Autodesk Fusion 360 part; units mm, degrees
(part 2 of 2)
sketch "Sketch25" plane through (0, 0, 0) normal (0, -1, 0) x (1, 0, 0)
  circle A0 centre (608.0806, 47.3768) radius 4
  circle A1 centre (290.245, 10.315) radius 1.632
  circle A2 centre (358.825, 49.685) radius 1.632
  circle A3 centre (290.245, 49.685) radius 1.632
  circle A4 centre (358.825, 10.315) radius 1.632
  line L0 (436.3768, 9) -> (436.3768, 7)
  line L1 (436.3768, 7) -> (431.3768, 7)
  line L2 (431.3768, 7) -> (431.3768, 9)
  line L3 (431.3768, 9) -> (436.3768, 9)
  line L4 (392.4, 53) -> (392.4, 51)
  line L5 (392.4, 51) -> (387.4, 51)
  line L6 (387.4, 51) -> (387.4, 53)
  line L7 (387.4, 53) -> (392.4, 53)
  line L8 (436.4, 53) -> (436.4, 51)
  line L9 (436.4, 51) -> (431.4, 51)
  line L10 (431.4, 51) -> (431.4, 53)
  line L11 (431.4, 53) -> (436.4, 53)
  line L12 (451.4, 22) -> (451.4, 17)
  line L13 (451.4, 17) -> (449.4, 17)
  line L14 (449.4, 17) -> (449.4, 22)
  line L15 (449.4, 22) -> (451.4, 22)
  line L16 (374.4, 22) -> (374.4, 17)
  line L17 (374.4, 17) -> (372.4, 17)
  line L18 (372.4, 17) -> (372.4, 22)
  line L19 (372.4, 22) -> (374.4, 22)
  line L20 (392.4, 7) -> (377.4, 7)
  line L21 (377.4, 7) -> (377.4, 47)
  arc A5 (378.4, 48) -> (377.4, 47) centre (378.4, 47) ccw
  line L22 (378.4, 48) -> (445.4, 48)
  arc A6 (446.4, 47) -> (445.4, 48) centre (445.4, 47) ccw
  line L23 (446.4, 47) -> (446.4, 13)
  arc A7 (445.4, 12) -> (446.4, 13) centre (445.4, 13) ccw
  line L24 (445.4, 12) -> (392.4, 12)
  line L25 (392.4, 12) -> (392.4, 7)
  line L26 (374.4, 43) -> (374.4, 38)
  line L27 (374.4, 38) -> (372.4, 38)
  line L28 (372.4, 38) -> (372.4, 43)
  line L29 (372.4, 43) -> (374.4, 43)
  line L30 (451.4, 43) -> (451.4, 38)
  line L31 (451.4, 38) -> (449.4, 38)
  line L32 (449.4, 38) -> (449.4, 43)
  line L33 (449.4, 43) -> (451.4, 43)
  line L34 (54.6452, 64.0786) -> (0.2658, 73.6672)
  arc A8 (0.2658, 73.6672) -> (15.4307, 51.4274) centre (30, 77.6521) ccw
  line L35 (15.4307, 51.4274) -> (47.2244, 33.7642)
  arc A9 (47.2244, 33.7642) -> (61.751, 29.989) centre (61.7937, 59.9889) ccw
  line L36 (61.751, 29.989) -> (121.5, 29.9038)
  arc A10 (121.5, 29.9038) -> (270.1218, 2.1743) centre (328.9822, 729.7974) ccw
  line L37 (270.1218, 2.1743) -> (297, 0)
  line L38 (297, 0) -> (481.4, 0)
  line L39 (481.4, 0) -> (481.4, 5)
  line L40 (481.4, 5) -> (486, 5)
  line L41 (486, 5) -> (486, 0)
  line L42 (486, 0) -> (638.7541, 27.9428)
  arc A11 (638.7541, 27.9428) -> (640.855, 36.8608) centre (637.8544, 32.8612) ccw
  line L43 (640.855, 36.8608) -> (618.013, 53.9974)
  arc A12 (618.013, 53.9974) -> (600.0096, 60) centre (600.0096, 30) ccw
  line L44 (600.0096, 60) -> (486, 60)
  line L45 (486, 60) -> (486, 55)
  line L46 (486, 55) -> (481.4, 55)
  line L47 (481.4, 55) -> (481.4, 60)
  line L48 (481.4, 60) -> (121.5429, 60)
  line L49 (121.5429, 60) -> (5.9649, 80.3795)
  arc A13 (5.9649, 80.3795) -> (0.931, 78.2208) centre (5.0967, 75.4555) ccw
  line L50 (0.931, 78.2208) -> (55.444, 68.6087)
  line L51 (55.444, 68.6087) -> (54.6452, 64.0786)
  line L52 (261, 60) -> (261, 2.9698)
  line L53 (270, 60) -> (274.6, 60)
  line L54 (274.6, 60) -> (274.6, 55)
  line L55 (274.6, 55) -> (270, 55)
  line L56 (270, 55) -> (270, 60)
  line L57 (247.4, 60) -> (252, 60)
  line L58 (252, 60) -> (252, 55)
  line L59 (252, 55) -> (247.4, 55)
  line L60 (247.4, 55) -> (247.4, 60)
  line L61 (224.8, 60) -> (229.4, 60)
  line L62 (229.4, 60) -> (229.4, 55)
  line L63 (229.4, 55) -> (224.8, 55)
  line L64 (224.8, 55) -> (224.8, 60)
  dimension "d204" = 225
  dimension "d205" = 5
  dimension "d206" = 4.6
  dimension "d207" = 9
  dimension "d208" = 9
  dimension "d209" = 18
  constraint coincident L48 L52.start
  constraint coincident A10 L52.end
  constraint perpendicular L48 L52
  constraint horizontal L53
  constraint vertical L54
  constraint horizontal L55
  constraint vertical L56
  constraint coincident L48 L53.start
  constraint horizontal L57
  constraint vertical L58
  constraint horizontal L59
  constraint vertical L60
  constraint coincident L48 L57.start
  constraint horizontal L61
  constraint vertical L62
  constraint horizontal L63
  constraint vertical L64
  constraint coincident L48 L61.start
  constraint equal L60 L62
  constraint equal L56 L60
  constraint equal L59 L63
  constraint equal L55 L59
  measures "d204" distance of L44.end L52.start
  measures "d205" distance of L61.start L63.end
  measures "d206" distance of L62.end L63.end
  measures "d207" distance of L52.start L53.start
  measures "d208" distance of L52.start L57.end
  measures "d209" distance of L57.start L61.end
extrude "Extrude14" cut sketch "Sketch25" against normal blind 10 contours L48 L61 L62 L63 L64 | L48 L57 L58 L59 L60 | L48 L53 L54 L55 L56
sketch "Sketch14" plane through (0, 0, 0) normal (0, -1, 0) x (1, 0, 0)
  circle A0 centre (608.0806, 47.3768) radius 4
  circle A1 centre (290.245, 10.315) radius 1.632
  circle A2 centre (358.825, 49.685) radius 1.632
  circle A3 centre (290.245, 49.685) radius 1.632
  circle A4 centre (358.825, 10.315) radius 1.632
  arc A5 (5.9649, 80.3795) -> (0.931, 78.2208) centre (5.0967, 75.4555) ccw
  arc A6 (0.2658, 73.6672) -> (15.4307, 51.4274) centre (30, 77.6521) ccw
  line L0 (15.4307, 51.4274) -> (47.2244, 33.7642)
  arc A7 (47.2244, 33.7642) -> (61.751, 29.989) centre (61.7937, 59.9889) ccw
  line L1 (61.751, 29.989) -> (121.5, 29.9038)
  arc A8 (121.5, 29.9038) -> (270.1218, 2.1743) centre (328.9822, 729.7974) ccw
  line L2 (270.1218, 2.1743) -> (297, 0)
  line L3 (297, 0) -> (481.4, 0)
  line L4 (481.4, 0) -> (481.4, 5)
  line L5 (481.4, 5) -> (486, 5)
  line L6 (486, 5) -> (486, 0)
  line L7 (486, 0) -> (638.7541, 27.9428)
  arc A9 (638.7541, 27.9428) -> (640.855, 36.8608) centre (637.8544, 32.8612) ccw
  line L8 (640.855, 36.8608) -> (618.013, 53.9974)
  arc A10 (618.013, 53.9974) -> (600.0096, 60) centre (600.0096, 30) ccw
  line L9 (600.0096, 60) -> (486, 60)
  line L10 (486, 60) -> (486, 55)
  line L11 (486, 55) -> (481.4, 55)
  line L12 (481.4, 55) -> (481.4, 60)
  line L13 (224.8, 60) -> (121.5429, 60)
  line L14 (121.5429, 60) -> (5.9649, 80.3795)
  line L15 (275.245, 44.697) -> (275.245, 13.8515)
  line L16 (146.3196, 50) -> (126.5286, 50)
  line L17 (126.5244, 47.0043) -> (126.5137, 39.5231)
  line L18 (145.6066, 31.7401) -> (196.4893, 23.3308)
  line L19 (121.5429, 60) -> (121.5, 29.9038)
  line L20 (275.245, 10.315) -> (290.245, 10.315)
  line L21 (77.8886, 34.966) -> (113.5071, 34.9152)
  line L22 (116.5114, 37.9109) -> (116.5245, 47.0988)
  line L23 (87.2027, 54.53) -> (28.389, 64.9004)
  line L24 (25.8981, 59.6835) -> (48.4796, 40.022)
  line L25 (54.2478, 30.9534) -> (54.2478, 71.8659)
  line L26 (15.4307, 51.4274) -> (15.4307, 78.7104)
  line L27 (496, 52) -> (496, 15.0573)
  line L28 (514.5755, 10.3102) -> (571.6338, 20.7477)
  line L29 (588.0806, 29.8203) -> (588.0806, 52)
  line L30 (588.0806, 55) -> (496, 55)
  line L31 (536.9832, 55) -> (499, 55)
  line L32 (544.4487, 55) -> (588.0806, 55)
  line L33 (290.245, 49.685) -> (345.825, 49.685)
  line L34 (358.825, 49.685) -> (358.825, 10.315)
  line L35 (358.825, 10.315) -> (303.245, 10.315)
  line L36 (290.245, 10.315) -> (290.245, 49.685)
  line L37 (315.5708, 49.4583) -> (348.825, 49.4583)
  line L38 (348.825, 46.685) -> (348.825, 17.6372)
  line L39 (334.6529, 10.0877) -> (300.245, 10.0877)
  line L40 (300.245, 13.315) -> (300.245, 43.0079)
  line L41 (130.7337, 36.7781) -> (147.5396, 44.2593)
  line L42 (144.7729, 37.3926) -> (163.7241, 46.7028)
  line L43 (166.5026, 46.6334) -> (198.4341, 28.9138)
  line L44 (179.9525, 44.4129) -> (215.683, 23.4364)
  line L45 (230.4442, 23.0758) -> (270.6997, 47.2684)
  line L46 (218.6893, 23.4182) -> (255.4279, 44.3948)
  line L47 (160.4357, 50) -> (170.4357, 50)
  line L48 (126.5071, 34.8967) -> (136.3733, 33.2661)
  line L49 (213.5872, 20.5051) -> (223.4534, 18.8745)
  line L50 (265.245, 50) -> (275.245, 50)
  line L51 (116.5071, 34.9109) -> (126.5071, 34.8967)
  line L52 (129.5244, 50) -> (160.4357, 50)
  line L53 (181.4714, 50) -> (253.9404, 50)
  line L54 (126.5071, 34.8967) -> (136.3733, 33.2661)
  line L55 (213.5872, 20.5051) -> (223.4534, 18.8745)
  line L56 (501.2833, 13.1114) -> (532.768, 50.0541)
  line L57 (511.7942, 15.2551) -> (541.0101, 48.0987)
  line L58 (554.2034, 49.6153) -> (583.2604, 27.4356)
  line L59 (545.1324, 48.4419) -> (572.9748, 26.0359)
  line L60 (496, 55) -> (530.4847, 55)
  line L61 (556.0237, 55) -> (585.0806, 55)
  line L62 (536.9832, 55) -> (547.1491, 55)
  line L63 (496, 6.9122) -> (506, 8.7415)
  line L64 (578.0806, 21.927) -> (588.0806, 23.7563)
  line L65 (112.7793, 50.009) -> (77.1477, 40.8719)
  line L66 (87.4269, 48.6696) -> (51.1948, 39.3785)
  line L67 (305.3143, 45.18) -> (336.7221, 15.2599)
  line L68 (313.5015, 44.2862) -> (343.7557, 15.465)
  arc A11 (28.389, 64.9004) -> (25.8981, 59.6835) centre (27.8681, 61.946) ccw
  arc A12 (48.4796, 40.022) -> (51.1948, 39.3785) centre (50.4496, 42.2845) ccw
  arc A13 (87.4269, 48.6696) -> (87.2027, 54.53) centre (86.6817, 51.5756) ccw
  arc A14 (77.1477, 40.8719) -> (77.8886, 34.966) centre (77.8929, 37.966) ccw
  arc A15 (116.5245, 47.0988) -> (112.7793, 50.009) centre (113.5245, 47.103) ccw
  arc A16 (113.5071, 34.9152) -> (116.5114, 37.9109) centre (113.5114, 37.9152) ccw
  arc A17 (129.5244, 50) -> (126.5244, 47.0043) centre (129.5244, 47) ccw
  arc A18 (126.5137, 39.5231) -> (130.7337, 36.7781) centre (129.5137, 39.5189) ccw
  arc A19 (147.5396, 44.2593) -> (146.3196, 50) centre (146.3196, 47) ccw
  arc A20 (166.5026, 46.6334) -> (163.7241, 46.7028) centre (165.047, 44.0102) ccw
  arc A21 (144.7729, 37.3926) -> (145.6066, 31.7401) centre (146.0957, 34.7) ccw
  arc A22 (196.4893, 23.3308) -> (198.4341, 28.9138) centre (196.9785, 26.2907) ccw
  arc A23 (181.4714, 50) -> (179.9525, 44.4129) centre (181.4714, 47) ccw
  arc A24 (215.683, 23.4364) -> (218.6893, 23.4182) centre (217.2018, 26.0235) ccw
  arc A25 (255.4279, 44.3948) -> (253.9404, 50) centre (253.9404, 47) ccw
  arc A26 (275.245, 44.697) -> (270.6997, 47.2684) centre (272.245, 44.697) ccw
  line L69 (231.5004, 17.5446) -> (271.7558, 10.8916)
  arc A27 (230.4442, 23.0758) -> (231.5004, 17.5446) centre (231.9895, 20.5045) ccw
  arc A28 (271.7558, 10.8916) -> (275.245, 13.8515) centre (272.245, 13.8515) ccw
  arc A29 (499, 55) -> (496, 52) centre (499, 52) ccw
  arc A30 (532.768, 50.0541) -> (530.4847, 55) centre (530.4847, 52) ccw
  arc A31 (496, 15.0573) -> (501.2833, 13.1114) centre (499, 15.0573) ccw
  arc A32 (545.1324, 48.4419) -> (541.0101, 48.0987) centre (543.2516, 46.1048) ccw
  arc A33 (511.7942, 15.2551) -> (514.5755, 10.3102) centre (514.0357, 13.2612) ccw
  arc A34 (556.0237, 55) -> (554.2034, 49.6153) centre (556.0237, 52) ccw
  arc A35 (588.0806, 52) -> (585.0806, 55) centre (585.0806, 52) ccw
  arc A36 (583.2604, 27.4356) -> (588.0806, 29.8203) centre (585.0806, 29.8203) ccw
  arc A37 (571.6338, 20.7477) -> (572.9748, 26.0359) centre (571.0939, 23.6987) ccw
  arc A38 (315.5708, 49.4583) -> (313.5015, 44.2862) centre (315.5708, 46.4583) ccw
  arc A39 (348.825, 46.685) -> (345.825, 49.685) centre (345.825, 46.685) ccw
  arc A40 (343.7557, 15.465) -> (348.825, 17.6372) centre (345.825, 17.6372) ccw
  arc A41 (334.6529, 10.0877) -> (336.7221, 15.2599) centre (334.6529, 13.0877) ccw
  arc A42 (300.245, 13.315) -> (303.245, 10.315) centre (303.245, 13.315) ccw
  arc A43 (305.3143, 45.18) -> (300.245, 43.0079) centre (303.245, 43.0079) ccw
  line L70 (436.3768, 9) -> (436.3768, 7)
  line L71 (436.3768, 7) -> (431.3768, 7)
  line L72 (431.3768, 7) -> (431.3768, 9)
  line L73 (431.3768, 9) -> (436.3768, 9)
  line L74 (392.4, 53) -> (392.4, 51)
  line L75 (392.4, 51) -> (387.4, 51)
  line L76 (387.4, 51) -> (387.4, 53)
  line L77 (387.4, 53) -> (392.4, 53)
  line L78 (436.4, 53) -> (436.4, 51)
  line L79 (436.4, 51) -> (431.4, 51)
  line L80 (431.4, 51) -> (431.4, 53)
  line L81 (431.4, 53) -> (436.4, 53)
  line L82 (451.4, 22) -> (451.4, 17)
  line L83 (451.4, 17) -> (449.4, 17)
  line L84 (449.4, 17) -> (449.4, 22)
  line L85 (449.4, 22) -> (451.4, 22)
  line L86 (374.4, 22) -> (374.4, 17)
  line L87 (374.4, 17) -> (372.4, 17)
  line L88 (372.4, 17) -> (372.4, 22)
  line L89 (372.4, 22) -> (374.4, 22)
  line L90 (392.4, 7) -> (377.4, 7)
  line L91 (377.4, 7) -> (377.4, 47)
  arc A44 (378.4, 48) -> (377.4, 47) centre (378.4, 47) ccw
  line L92 (378.4, 48) -> (445.4, 48)
  arc A45 (446.4, 47) -> (445.4, 48) centre (445.4, 47) ccw
  line L93 (446.4, 47) -> (446.4, 13)
  arc A46 (445.4, 12) -> (446.4, 13) centre (445.4, 13) ccw
  line L94 (445.4, 12) -> (392.4, 12)
  line L95 (392.4, 12) -> (392.4, 7)
  line L96 (374.4, 43) -> (374.4, 38)
  line L97 (374.4, 38) -> (372.4, 38)
  line L98 (372.4, 38) -> (372.4, 43)
  line L99 (372.4, 43) -> (374.4, 43)
  line L100 (451.4, 43) -> (451.4, 38)
  line L101 (451.4, 38) -> (449.4, 38)
  line L102 (449.4, 38) -> (449.4, 43)
  line L103 (449.4, 43) -> (451.4, 43)
  line L104 (54.6452, 64.0786) -> (0.2658, 73.6672)
  line L105 (0.931, 78.2208) -> (55.444, 68.6087)
  line L106 (55.444, 68.6087) -> (54.6452, 64.0786)
  line L107 (224.8, 55) -> (224.8, 60)
  line L108 (481.4, 60) -> (274.6, 60)
  line L109 (274.6, 60) -> (274.6, 55)
  line L110 (274.6, 55) -> (270, 55)
  line L111 (270, 55) -> (270, 60)
  line L112 (270, 60) -> (252, 60)
  line L113 (252, 60) -> (252, 55)
  line L114 (252, 55) -> (247.4, 55)
  line L115 (247.4, 55) -> (247.4, 60)
  line L116 (247.4, 60) -> (229.4, 60)
  line L117 (229.4, 60) -> (229.4, 55)
  line L118 (229.4, 55) -> (224.8, 55)
  dimension "d128" = 5
  dimension "d131" = 15
  dimension "d134" = 5
  dimension "d138" = 10
  dimension "d139" = 20
  dimension "d141" = 5
  dimension "d142" = 5
  dimension "d143" = 10
  dimension "d144" = 10
  dimension "d149" = 10
  dimension "d150" = 5
  dimension "d154" = 10
  dimension "d155" = 10
  dimension "d156" = 5
  dimension "d158" = 5
  dimension "d159" = 3
  dimension "d160" = 3
  dimension "d161" = 3
  dimension "d162" = 3
  dimension "d163" = 3
  dimension "d164" = 3
  dimension "d165" = 3
  dimension "d166" = 3
  dimension "d167" = 3
  dimension "d168" = 3
  dimension "d169" = 3
  dimension "d170" = 3
  dimension "d171" = 3
  dimension "d172" = 3
  dimension "d173" = 3
  dimension "d174" = 3
  dimension "d175" = 3
  dimension "d176" = 3
  dimension "d177" = 3
  dimension "d178" = 3
  dimension "d179" = 3
  dimension "d180" = 3
  dimension "d181" = 3
  dimension "d182" = 3
  dimension "d183" = 3
  dimension "d184" = 3
  dimension "d185" = 3
  dimension "d186" = 3
  dimension "d187" = 3
  dimension "d188" = 3
  dimension "d189" = 3
  dimension "d190" = 3
  dimension "d191" = 3
  constraint coincident L16 L47.start
  constraint coincident L13.end L14.start
  constraint coincident L1.end A8.start
  constraint parallel L17 L19
  constraint parallel L13 L16
  constraint coincident A1.centre L20.end
  constraint parallel L13 L20
  constraint parallel L19 L22
  constraint parallel L1 L21
  constraint midpoint A7 L25.start
  constraint coincident L14 L25.end
  constraint vertical L25
  constraint coincident A6.end L0.start
  constraint coincident L14 L26.end
  constraint vertical L26
  constraint parallel L12 L27
  constraint parallel L12 L29
  constraint perpendicular L27 L30
  constraint coincident L30 L31.start
  constraint perpendicular L29 L32
  constraint parallel L7 L28
  constraint horizontal L33
  constraint vertical L34
  constraint horizontal L35
  constraint vertical L36
  constraint coincident A4.centre L34.end
  constraint coincident A3.centre L33.start
  constraint horizontal L37
  constraint vertical L38
  constraint horizontal L39
  constraint vertical L40
  constraint coincident L18 L48.end
  constraint coincident L18 L49.start
  constraint coincident L18 L49.end
  constraint coincident L16 L50.start
  constraint horizontal L47
  constraint perpendicular L17 L51
  constraint perpendicular L15 L20
  constraint parallel L16 L53
  constraint equal L47 L50
  constraint equal L49 L50
  constraint parallel L48 L54
  constraint parallel L49 L55
  constraint equal L54 L55
  constraint coincident L28 L63.end
  constraint coincident L32 L62.end
  constraint coincident L28 L64.start
  constraint equal L62 L63
  constraint equal L63 L64
  constraint parallel L65 L66
  constraint parallel L67 L68
  constraint tangent L24 A11
  constraint tangent L23 A11
  constraint tangent L24 A12
  constraint tangent L66 A12
  constraint tangent L66 A13
  constraint tangent L23 A13
  constraint tangent L65 A14
  constraint tangent L21 A14
  constraint tangent L22 A15
  constraint tangent L65 A15
  constraint coincident L51.start L21
  constraint coincident L51.start L22
  constraint tangent L21 A16
  constraint tangent L22 A16
  constraint coincident L16.end L17
  constraint coincident L16.end L52
  constraint tangent L17 A17
  constraint tangent L52 A17
  constraint coincident L48.start L17
  constraint coincident L48.start L41
  constraint tangent L17 A18
  constraint tangent L41 A18
  constraint coincident L50.end L16
  constraint coincident L47.start L41
  constraint tangent L16 A19
  constraint tangent L41 A19
  constraint coincident L47.end L42
  constraint coincident L47.start L43
  constraint tangent L42 A20
  constraint tangent L43 A20
  constraint coincident L48.end L42
  constraint coincident L48.start L18
  constraint tangent L42 A21
  constraint tangent L18 A21
  constraint coincident L49.start L43
  constraint coincident L20.start L18
  constraint tangent L43 A22
  constraint tangent L18 A22
  constraint coincident L47.end L44
  constraint tangent L53 A23
  constraint tangent L44 A23
  constraint coincident L49.end L44
  constraint coincident L49.start L46
  constraint tangent L44 A24
  constraint tangent L46 A24
  constraint coincident L50.start L46
  constraint coincident L50.start L53
  constraint tangent L46 A25
  constraint tangent L53 A25
  constraint coincident L50.end L45
  constraint coincident L50.end L15
  constraint tangent L45 A26
  constraint tangent L15 A26
  constraint coincident L49.end L45
  constraint coincident L49.end L69
  constraint tangent L45 A27
  constraint tangent L69 A27
  constraint coincident L20.start L69
  constraint coincident L20.start L15
  constraint tangent L69 A28
  constraint tangent L15 A28
  constraint coincident L30.end L31
  constraint coincident L30.end L27
  constraint tangent L31 A29
  constraint tangent L27 A29
  constraint coincident L31.start L60
  constraint coincident L31.start L56
  constraint tangent L60 A30
  constraint tangent L56 A30
  constraint coincident L63.start L56
  constraint coincident L63.start L27
  constraint tangent L56 A31
  constraint tangent L27 A31
  constraint coincident L62.end L57
  constraint coincident L31.start L59
  constraint tangent L57 A32
  constraint tangent L59 A32
  constraint coincident L63.end L57
  constraint coincident L63.start L28
  constraint tangent L57 A33
  constraint tangent L28 A33
  constraint coincident L62.end L58
  constraint coincident L62.end L61
  constraint tangent L58 A34
  constraint tangent L61 A34
  constraint coincident L30.start L61
  constraint coincident L30.start L29
  constraint tangent L61 A35
  constraint tangent L29 A35
  constraint coincident L64.end L58
  constraint coincident L64.end L29
  constraint tangent L58 A36
  constraint tangent L29 A36
  constraint coincident L64.start L59
  constraint coincident L64.end L28
  constraint tangent L59 A37
  constraint tangent L28 A37
  constraint tangent L37 A38
  constraint tangent L68 A38
  constraint coincident A2.centre L33
  constraint coincident L37.end L38
  constraint tangent L33 A39
  constraint tangent L38 A39
  constraint tangent L68 A40
  constraint tangent L38 A40
  constraint tangent L67 A41
  constraint tangent L39 A41
  constraint coincident A1.centre L35
  constraint coincident L39.end L40
  constraint tangent L35 A42
  constraint tangent L40 A42
  constraint tangent L40 A43
  constraint tangent L67 A43
  measures "d128" distance of L17 L19
  measures "d131" distance of A3.centre L15
  measures "d134" distance of L19 L22
  measures "d138" distance of L10.end L27
  measures "d139" distance of A0.centre L29
  measures "d141" distance of L9 L30
  measures "d142" distance of L7 L28
  measures "d143" distance of L36 L40
  measures "d144" distance of L34 L38
  measures "d149" distance of L13 L16
  measures "d150" distance of L1.end L51
  measures "d154" distance of L48.start L48.end
  measures "d155" horizontal distance of L63.start L63.end
  measures "d156" distance of L65 L66
  measures "d158" distance of L67 L68
  measures "d159" radius of A11
  measures "d160" radius of A12
  measures "d161" radius of A13
  measures "d162" radius of A14
  measures "d163" radius of A15
  measures "d164" radius of A16
  measures "d165" radius of A17
  measures "d166" radius of A18
  measures "d167" radius of A19
  measures "d168" radius of A20
  measures "d169" radius of A21
  measures "d170" radius of A22
  measures "d171" radius of A23
  measures "d172" radius of A24
  measures "d173" radius of A25
  measures "d174" radius of A26
  measures "d175" radius of A27
  measures "d176" radius of A28
  measures "d177" radius of A29
  measures "d178" radius of A30
  measures "d179" radius of A31
  measures "d180" radius of A32
  measures "d181" radius of A33
  measures "d182" radius of A34
  measures "d183" radius of A35
  measures "d184" radius of A36
  measures "d185" radius of A37
  measures "d186" radius of A38
  measures "d187" radius of A39
  measures "d188" radius of A40
  measures "d189" radius of A41
  measures "d190" radius of A42
  measures "d191" radius of A43
extrude "Extrude11" cut sketch "Sketch14" against normal blind 20 contours L23 L24 L25 L66 A11 A12 | L23 L25 L66 A13 | L15 L45 A26 L69 A27 A28 | L16 L17 L41 L52 A17 A18 A19 | L18 L42 L43 A20 A21 A22 | L21 L22 L65 A14 A15 A16 | L27 L30 L31 L56 L60 A29 A30 A31 | L28 L57 L59 A32 A33 A37 | L29 L30 L32 L58 L61 A34 A35 A36 | L35 L40 L67 A41 A42 A43 | L37 L38 L68 A38 A39 A40 | L44 L46 L53 A23 A24 A25
ref_plane "WorkPlane1" through (121.5191, 2.25, 43.2708) normal (0.999999, 0, -0.001425) x (-0.001425, 0, -0.999999)
equation "d34 = ( 27 * 4.5 ) * 1 mm"
equation "d37 = ( 27 * 11 ) * 1 mm"
equation "d38 = ( 27 * 18 ) * 1 mm"

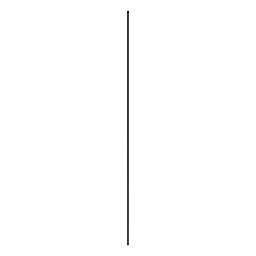
design "small spar short"
Autodesk Fusion 360 part; units mm, degrees
sketch "Sketch1" plane through (0, 0, 0) normal (0, 0, 1) x (1, 0, 0)
  circle A0 centre (0, 0) radius 1
  dimension "d1" = 2
  constraint coincident A0.centre origin
  measures "d1" diameter of A0
extrude "Extrude1" add sketch "Sketch1" along normal blind 322

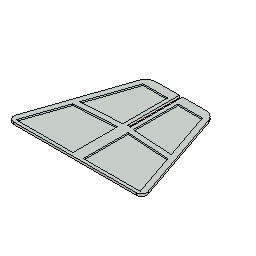
design "Tail Wing"
Autodesk Fusion 360 part; units mm, degrees
sketch "Sketch1" plane through (0, 0, 0) normal (0, 0, 1) x (1, 0, 0)
  line L0 (0, 0) -> (120, 0)
  line L1 (120, 0) -> (120, 120)
  line L2 (120, 120) -> (0, 120)
  line L3 (0, 120) -> (0, 0)
  dimension "d1" = 120
  constraint horizontal L0
  constraint vertical L1
  constraint horizontal L2
  constraint vertical L3
  constraint coincident L0.start L3.end
  constraint equal L0 L3
  measures "d1" distance of L1 L3
sketch "Sketch2" plane through (0, 0, 0) normal (0, 0, 1) x (1, 0, 0)
  line L0 (120.1825, 14.3012) -> (85.1178, 116.8012)
  line L1 (85.1178, 116.8012) -> (58.9029, 116.8012)
  line L2 (58.9029, 116.8012) -> (58.9029, 14.3012)
  line L3 (58.9029, 14.3012) -> (120.1825, 14.3012)
  line L4 (58.9029, 108.8012) -> (82.5701, 108.8012)
  line L5 (82.5701, 108.8012) -> (113.8718, 17.3012)
  line L6 (113.8718, 17.3012) -> (58.9029, 17.3012)
  line L7 (98.2209, 63.0512) -> (58.9029, 65.5512)
  line L8 (99.9346, 58.042) -> (58.9029, 60.6509)
  line L9 (58.9029, 116.8012) -> (48.9029, 116.8012)
  line L10 (48.9029, 116.8012) -> (48.9029, 14.3012)
  line L11 (48.9029, 14.3012) -> (58.9029, 14.3012)
  line L12 (58.9029, 14.3012) -> (58.9029, 116.8012)
  line L13 (53.9029, 116.8012) -> (53.9029, 14.3012)
  line L14 (48.9029, 108.8012) -> (25.2358, 108.8012)
  line L15 (22.6881, 116.8012) -> (48.9029, 116.8012)
  line L16 (-12.3766, 14.3012) -> (22.6881, 116.8012)
  line L17 (25.2358, 108.8012) -> (-6.0659, 17.3012)
  line L18 (9.585, 63.0512) -> (48.9029, 65.5512)
  line L19 (7.8713, 58.042) -> (48.9029, 60.6509)
  line L20 (-6.0659, 17.3012) -> (48.9029, 17.3012)
  line L21 (48.9029, 14.3012) -> (-12.3766, 14.3012)
  line L22 (48.9029, 14.3012) -> (48.9029, 116.8012)
  line L23 (58.9029, 14.3012) -> (48.9029, 14.3012)
  line L24 (48.9029, 116.8012) -> (58.9029, 116.8012)
  line L25 (48.9029, 17.3012) -> (48.9029, 14.3012)
  point P0 (120.1825, 14.3012)
  point P1 (53.9029, 14.3012)
  dimension "d2" = 3
  dimension "d3" = 5
  dimension "d4" = 8
  dimension "d5" = 10
  dimension "d18" = 102.5
  constraint coincident P0 L0.start
  constraint horizontal L1
  constraint perpendicular L1 L2
  constraint perpendicular L2 L3
  constraint coincident L2 L4.start
  constraint perpendicular L2 L4
  constraint parallel L0 L5
  constraint coincident L2 L6.end
  constraint perpendicular L2 L6
  constraint midpoint L5 L7.start
  constraint midpoint L2 L7.end
  constraint coincident L5 L8.start
  constraint coincident L2 L8.end
  constraint parallel L7 L8
  constraint horizontal L9
  constraint vertical L10
  constraint horizontal L11
  constraint vertical L12
  constraint midpoint L9 L13.start
  constraint midpoint L11 P1
  constraint symmetric P0 L13 L16.start
  constraint symmetric L0.end L13 L15.start
  constraint symmetric L1.end L13 L9.end
  constraint symmetric L2.end L13 L10.end
  constraint symmetric L4.start L13 L14.start
  constraint symmetric L4.end L13 L14.end
  constraint symmetric L5.end L13 L17.end
  constraint symmetric L6.end L13 L20.end
  constraint symmetric L7.start L13 L18.start
  constraint symmetric L7.end L13 L18.end
  constraint symmetric L8.start L13 L19.start
  constraint symmetric L8.end L13 L19.end
  constraint symmetric L9.end L13 L1.end
  constraint symmetric L10.end L13 L2.end
  constraint symmetric P1 L13 L13.end
  constraint coincident L10.end L11.start
  measures "d2" distance of L3 L6
  measures "d3" distance of L0 L5
  measures "d4" distance of L1 L4
  measures "d5" distance of L10 L12
  measures "d18" distance of L15 L21
extrude "Extrude1" add sketch "Sketch2" along normal blind 3.175 contours L0 L1 L2 L3 L4 L5 L6 L12 | L2 L9 L11 L12 L13 L23 L24 | L9 L10 L11 L13 L22 L23 L24 L25 | L2 L5 L7 L8 L12 | L10 L14 L15 L16 L17 L20 L21 L22 L25 | L10 L17 L18 L19 L22
extrude "Extrude2" add sketch "Sketch2" along normal blind 1 contours L2 L5 L6 L8 L12 | L2 L4 L5 L7 L12 | L10 L17 L19 L20 L22 | L10 L14 L17 L18 L22
fillet "Fillet1" radius 10 1 edges at (85.1178, 116.8012, 1.5875)
fillet "Fillet2" radius 10 1 edges at (22.6881, 116.8012, 1.5875)
fillet "Fillet3" radius 5 1 edges at (120.1825, 14.3012, 1.5875)
fillet "Fillet5" radius 5 1 edges at (-12.3766, 14.3012, 1.5875)
scale "Scale1" factors (1.5, 1.5, 1) about (48.9029, 65.5512, 1) bodies 1
sketch "Sketch5" plane through (0, 0, 3.175) normal (0, 0, 1) x (-1, 0, 0)
  arc A0 (39.6202, 1.3962) -> (32.524, 11.3238) centre (32.524, 3.8238) ccw
  line L0 (32.524, 11.3238) -> (-145.3299, 11.3238)
  arc A1 (-145.3299, 11.3238) -> (-152.4261, 1.3962) centre (-145.3299, 3.8238) ccw
  line L1 (-152.4261, 1.3962) -> (-106.6957, -132.2814)
  arc A2 (-106.6957, -132.2814) -> (-92.5032, -142.4262) centre (-92.5032, -127.4262) ccw
  line L2 (-92.5032, -142.4262) -> (-20.3027, -142.4262)
  arc A3 (-20.3027, -142.4262) -> (-6.1102, -132.2814) centre (-20.3027, -127.4262) ccw
  line L3 (-6.1102, -132.2814) -> (39.6202, 1.3962)
  line L4 (-99.4036, -130.4262) -> (-122.8799, -61.8012)
  line L5 (-122.8799, -61.8012) -> (-63.9029, -65.5512)
  line L6 (-63.9029, -65.5512) -> (-63.9029, -130.4262)
  line L7 (-63.9029, -130.4262) -> (-99.4036, -130.4262)
  line L8 (33.5503, 6.8238) -> (12.6445, -54.2873)
  line L9 (12.6445, -54.2873) -> (-48.9029, -58.2008)
  line L10 (-48.9029, -58.2008) -> (-48.9029, 6.8238)
  line L11 (-48.9029, 6.8238) -> (33.5503, 6.8238)
  line L12 (-63.9029, -58.2008) -> (-125.4504, -54.2873)
  line L13 (-125.4504, -54.2873) -> (-146.3562, 6.8238)
  line L14 (-146.3562, 6.8238) -> (-63.9029, 6.8238)
  line L15 (-63.9029, 6.8238) -> (-63.9029, -58.2008)
  line L16 (-48.9029, -65.5512) -> (10.074, -61.8012)
  line L17 (10.074, -61.8012) -> (-13.4023, -130.4262)
  line L18 (-13.4023, -130.4262) -> (-48.9029, -130.4262)
  line L19 (-48.9029, -130.4262) -> (-48.9029, -65.5512)
  line L20 (-54.1029, -142.4262) -> (-58.7029, -142.4262)
  line L21 (-58.7029, -142.4262) -> (-58.7029, -67.4262)
  line L22 (-58.7029, -67.4262) -> (-54.1029, -67.4262)
  line L23 (-54.1029, -67.4262) -> (-54.1029, -142.4262)
  line L24 (-54.1029, -132.8434) -> (-48.9029, -132.8434)
  line L25 (-58.7029, -133.3407) -> (-63.9029, -133.3407)
  dimension "d28" = 4.6
  dimension "d29" = 75
  constraint horizontal L20
  constraint vertical L21
  constraint horizontal L22
  constraint vertical L23
  constraint coincident L2 L20.start
  constraint coincident L23 L24.start
  constraint coincident L19 L24.end
  constraint perpendicular L19 L24
  constraint coincident L21 L25.start
  constraint coincident L6 L25.end
  constraint perpendicular L6 L25
  constraint equal L24 L25
  measures "d28" distance of L21 L23
  measures "d29" distance of L20.start L22.end
extrude "Extrude4" cut sketch "Sketch5" against normal blind 10 contours L2 L20 L21 L22 L23
sketch "Sketch7" plane through (0, 0, 3.175) normal (0, 0, 1) x (-1, 0, 0)
  line L0 (-54.1029, -67.4262) -> (-54.1029, -142.4262)
  line L1 (-54.1029, -142.4262) -> (-20.3027, -142.4262)
  arc A0 (-20.3027, -142.4262) -> (-6.1102, -132.2814) centre (-20.3027, -127.4262) ccw
  line L2 (-6.1102, -132.2814) -> (39.6202, 1.3962)
  arc A1 (39.6202, 1.3962) -> (32.524, 11.3238) centre (32.524, 3.8238) ccw
  line L3 (32.524, 11.3238) -> (-145.3299, 11.3238)
  arc A2 (-145.3299, 11.3238) -> (-152.4261, 1.3962) centre (-145.3299, 3.8238) ccw
  line L4 (-152.4261, 1.3962) -> (-106.6957, -132.2814)
  arc A3 (-106.6957, -132.2814) -> (-92.5032, -142.4262) centre (-92.5032, -127.4262) ccw
  line L5 (-92.5032, -142.4262) -> (-58.7029, -142.4262)
  line L6 (-58.7029, -142.4262) -> (-58.7029, -67.4262)
  line L7 (-58.7029, -67.4262) -> (-54.1029, -67.4262)
  line L8 (-99.4036, -130.4262) -> (-122.8799, -61.8012)
  line L9 (-122.8799, -61.8012) -> (-63.9029, -65.5512)
  line L10 (-63.9029, -65.5512) -> (-63.9029, -130.4262)
  line L11 (-63.9029, -130.4262) -> (-99.4036, -130.4262)
  line L12 (-63.9029, -58.2008) -> (-125.4504, -54.2873)
  line L13 (-125.4504, -54.2873) -> (-146.3562, 6.8238)
  line L14 (-146.3562, 6.8238) -> (-63.9029, 6.8238)
  line L15 (-63.9029, 6.8238) -> (-63.9029, -58.2008)
  line L16 (33.5503, 6.8238) -> (12.6445, -54.2873)
  line L17 (12.6445, -54.2873) -> (-48.9029, -58.2008)
  line L18 (-48.9029, -58.2008) -> (-48.9029, 6.8238)
  line L19 (-48.9029, 6.8238) -> (33.5503, 6.8238)
  line L20 (-48.9029, -65.5512) -> (10.074, -61.8012)
  line L21 (10.074, -61.8012) -> (-13.4023, -130.4262)
  line L22 (-13.4023, -130.4262) -> (-48.9029, -130.4262)
  line L23 (-48.9029, -130.4262) -> (-48.9029, -65.5512)

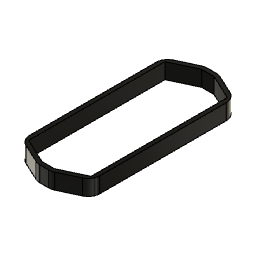
design "ziptie"
Autodesk Fusion 360 part; units mm, degrees
sketch "Sketch1" plane through (0, 0, 0) normal (0, 0, 1) x (1, 0, 0)
  line L0 (0, 0) -> (16, 0)
  line L1 (16, 0) -> (16, 41)
  line L2 (16, 41) -> (0, 41)
  line L3 (0, 41) -> (0, 0)
  line L4 (6.4125, 41) -> (9.5875, 41)
  line L5 (9.5875, 41) -> (9.5875, 0)
  line L6 (9.5875, 0) -> (6.4125, 0)
  line L7 (6.4125, 0) -> (6.4125, 41)
  line L8 (0, 20.5) -> (6.4125, 20.5)
  line L9 (9.5875, 20.5) -> (16, 20.5)
  line L10 (0, 38) -> (16, 38)
  line L11 (0, 3) -> (16, 3)
  line L12 (16, 3) -> (16, 0)
  line L13 (16, 38) -> (16, 41)
  line L14 (6.4125, 41) -> (0, 38)
  line L15 (0, 20.5) -> (0, 3)
  line L16 (6.4125, 0) -> (9.5875, 0)
  line L17 (16, 3) -> (16, 20.5)
  line L18 (16, 38) -> (9.5875, 41)
  line L19 (6.4125, 41) -> (9.5875, 41)
  line L20 (9.5875, 41) -> (9.5875, 42)
  line L21 (9.5875, 42) -> (6.4125, 42)
  line L22 (6.4125, 42) -> (6.4125, 41)
  line L23 (16, 38) -> (17, 38)
  line L24 (17, 38) -> (17, 2.9976)
  line L25 (17, 2.9976) -> (16, 2.9976)
  line L26 (16, 2.9976) -> (16, 38)
  line L27 (6.4125, 0) -> (9.5471, 0)
  line L28 (9.5471, 0) -> (9.5471, -1)
  line L29 (9.5471, -1) -> (6.4125, -1)
  line L30 (6.4125, -1) -> (6.4125, 0)
  line L31 (0, 3) -> (-1, 3)
  line L32 (-1, 3) -> (-1, 38.0102)
  line L33 (-1, 38.0102) -> (0, 38.0102)
  line L34 (0, 38.0102) -> (0, 3)
  line L35 (0, 38) -> (6.4125, 41)
  line L36 (6.4125, 41) -> (5.9887, 41.9058)
  line L37 (5.9887, 41.9058) -> (-0.4238, 38.9058)
  line L38 (-0.4238, 38.9058) -> (0, 38)
  line L39 (9.5875, 41) -> (16, 38)
  line L40 (16, 38) -> (16.4238, 38.9058)
  line L41 (16.4238, 38.9058) -> (10.0113, 41.9058)
  line L42 (10.0113, 41.9058) -> (9.5875, 41)
  line L43 (16, 3) -> (9.5875, 0)
  line L44 (9.5875, 0) -> (10.0113, -0.9058)
  line L45 (10.0113, -0.9058) -> (16.4238, 2.0942)
  line L46 (16.4238, 2.0942) -> (16, 3)
  line L47 (0, 3) -> (6.4125, 0)
  line L48 (6.4125, 0) -> (5.9887, -0.9058)
  line L49 (5.9887, -0.9058) -> (-0.4238, 2.0942)
  line L50 (-0.4238, 2.0942) -> (0, 3)
  line L51 (-1, 38.0102) -> (-0.4238, 38.9058)
  line L52 (5.9887, 41.9058) -> (6.4125, 42)
  line L53 (9.5875, 42) -> (10.0113, 41.9058)
  line L54 (16.4238, 38.9058) -> (17, 38)
  line L55 (17, 2.9976) -> (16.4238, 2.0942)
  line L56 (6.4125, -1) -> (5.9887, -0.9058)
  line L57 (9.5471, -1) -> (10.0113, -0.9058)
  line L58 (-0.4238, 2.0942) -> (-1, 3)
  dimension "d1" = 16
  dimension "d2" = 41
  dimension "d3" = 3.175
  dimension "d4" = 3
  dimension "d6" = 1
  constraint horizontal L0
  constraint vertical L1
  constraint horizontal L2
  constraint vertical L3
  constraint coincident L0.start L3.end
  constraint horizontal L4
  constraint vertical L5
  constraint horizontal L6
  constraint vertical L7
  constraint coincident L0 L5.end
  constraint coincident L2 L4.start
  constraint midpoint L3 L8.start
  constraint midpoint L7 L8.end
  constraint midpoint L5 L9.start
  constraint midpoint L1 L9.end
  constraint equal L8 L9
  constraint coincident L3 L10.start
  constraint coincident L1 L10.end
  constraint perpendicular L1 L10
  constraint coincident L3 L11.start
  constraint coincident L1 L11.end
  constraint perpendicular L1 L11
  constraint perpendicular L0 L12
  constraint equal L12 L13
  constraint horizontal L19
  constraint vertical L20
  constraint horizontal L21
  constraint vertical L22
  constraint horizontal L23
  constraint vertical L24
  constraint horizontal L25
  constraint vertical L26
  constraint horizontal L27
  constraint vertical L28
  constraint horizontal L29
  constraint vertical L30
  constraint horizontal L31
  constraint vertical L32
  constraint horizontal L33
  constraint vertical L34
  constraint equal L20 L23
  constraint equal L23 L28
  constraint equal L28 L31
  constraint perpendicular L35 L36
  constraint parallel L35 L37
  constraint parallel L36 L38
  constraint perpendicular L39 L40
  constraint parallel L39 L41
  constraint parallel L40 L42
  constraint parallel L18 L39
  constraint perpendicular L43 L44
  constraint parallel L43 L45
  constraint parallel L44 L46
  constraint perpendicular L47 L48
  constraint parallel L47 L49
  constraint parallel L48 L50
  constraint equal L33 L38
  constraint equal L23 L40
  constraint equal L25 L46
  constraint equal L31 L50
  constraint coincident L4.end L20
  measures "d1" distance of L1 L3
  measures "d2" distance of L0 L2
  measures "d3" distance of L5 L7
  measures "d4" distance of L2 L10
  measures "d6" distance of L2 L21
extrude "Extrude1" add sketch "Sketch1" along normal blind 4 contours L0 L48 L49 | L0 L6 L16 L27 L28 L29 L30 | L0 L3 L47 L49 | L30 L48 L56 | L0 L6 L16 L28 L44 L57 | L3 L15 L31 L32 L33 L34 L38 | L31 L50 L58 | L3 L49 L50 | L0 L1 L12 L43 L45 | L0 L44 L45 | L1 L12 L45 L46 | L1 L17 L23 L24 L25 L26 | L25 L46 L55 | L2 L3 L14 L34 L35 L37 | L33 L38 L51 | L2 L4 L19 L20 L21 L22 | L22 L36 L52 | L2 L36 L37 | L3 L33 L37 L38 | L1 L2 L13 L18 L39 L41 | L23 L40 L54 | L1 L13 L40 L41 | L2 L41 L42 | L20 L42 L53
fillet "Fillet1" radius 3 16 edges at (9.5875, 42, 2) (10.0113, 41.9058, 2) (6.4125, 42, 2) (5.9887, 41.9058, 2) (-0.4238, 38.9058, 2) (-1, 38.0102, 2) (-1, 3, 2) (-0.4238, 2.0942, 2) (5.9887, -0.9058, 2) (6.4125, -1, 2) (9.5471, -1, 2) (10.0113, -0.9058, 2) (16.4238, 2.0942, 2) (17, 2.9976, 2) (17, 38, 2) (16.4238, 38.9058, 2)
